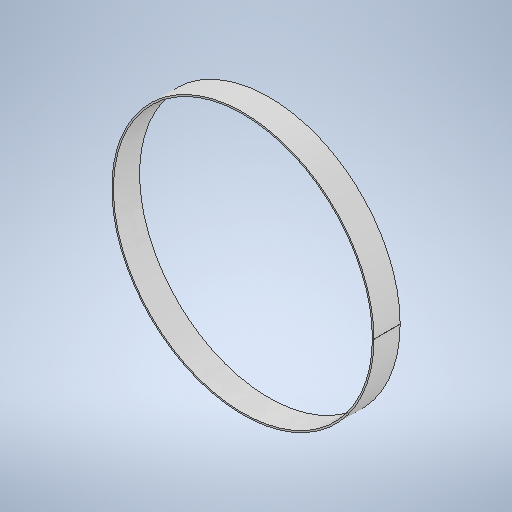
# Autodesk Inventor part: MSC 035 ring
Saved by Autodesk Inventor 2025 (Build 290162010, 162A)
## iProperties
Created: 2024-06-19
Part Number: MSC 035 ring
Material: Stainless Steel
Document SubType Name: Sheet Metal
Designer: pokla
Density: 8 g/cm^3
Flat Pattern Width: 155.981 cm
Flat Pattern Length: 5 cm
Flat Pattern Area: 779.904 cm^2
Sheet Metal Rule: AISI304 3mm Die 32
Sheet Metal Width: 1559,807 mm
Sheet Metal Length: 50,000 mm
Sheet Metal Area: 77990,359 mm^2
Appearance: Default
Author: pokla
Autodesk Inventor part; units mm, degrees
ref_plane "YZ Plane" through (0, 0, 0) normal (1, 0, 0) x (0, 1, 0)
ref_plane "XZ Plane" through (0, 0, 0) normal (0, 1, 0) x (-1, 0, 0)
ref_plane "XY Plane" through (0, 0, 0) normal (0, 0, 1) x (1, 0, 0)
sketch "Sketch3" plane through (0, 0, 0) normal (0, 0, 1) x (1, 0, 0)
  line L0 (-250, 25) -> (-247, 25)
  line L1 (-247, 25) -> (-247, -25)
  line L2 (-247, -25) -> (-250, -25)
  line L3 (-250, -25) -> (-250, 25)
  line L4 (0, -35) -> (0, 35) projected
  point P0 (0, 0)
  point P1 (-250, 0)
  dimension "d1" = 3
  dimension "d2" = 50
  dimension "d3" = 250
  constraints: 8 end point, 2 parallel, 1 horizontal, 1 horizontal alignment, 1 midpoint, 1 perpendicular
  measures "d1" distance of L0.start L0.end
  measures "d2" distance of L2.end L0.start
  measures "d3" distance of point (0, 0) point (-250, 0)
revolve "Revolution1" add sketch "Sketch3" angle 359.9 mid plane about axis through (0, -10, 0) along (0, 1, 0)
equation "\"BendReliefWidth\" = Thickness"
equation "\"BendReliefDepth\" = 0.5 * Thickness"
equation "\"CornerReliefSize\" = 4 * Thickness"
equation "\"MinimumRemnant\" = 2 * Thickness"
equation "\"TransitionRadius\" = BendRadius"
equation "\"JacobiRadiusSize\" = BendRadius"
equation "\"GapSize\" = Thickness"
equation "\"Thickness\" = 3"
equation "\"BendRadius\" = 5"
body "Solid1"
